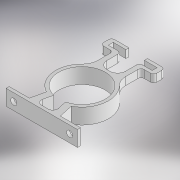
# Autodesk Inventor part: DefaultMotorMount
Saved by Autodesk Inventor 2018.2 (Build 222227000, 227)
## iProperties
Created: 2018-03-31
Part Number: DefaultMotorMount
Material: ABS Plastic
Document SubType Name: Modeling
Designer: Muchen He
Density: 1.06 g/cm^3
Appearance: Smooth - White
Author: Muchen He
Autodesk Inventor part; units mm, degrees
ref_plane "YZ Plane" through (0, 0, 0) normal (1, 0, 0) x (0, 1, 0)
ref_plane "XZ Plane" through (0, 0, 0) normal (0, 1, 0) x (-1, 0, 0)
ref_plane "XY Plane" through (0, 0, 0) normal (0, 0, 1) x (1, 0, 0)
sketch "Sketch1" plane through (0, 0, 0) normal (0, 0, 1) x (1, 0, 0)
  line L0 (0, 0) -> (23, 0)
  line L1 (23, 0) -> (23, 2)
  line L2 (23, 2) -> (10, 2)
  line L3 (10, 2) -> (8, 11)
  line L4 (0, 0) -> (0, 26) construction
  arc A0 (8, 11) -> (0, 43) centre (0, 26) ccw
  line L5 (18, 2) -> (18, 0) construction
  arc A1 (3.794, 11.4878) -> (0, 41) centre (0, 26) ccw
  line L6 (3.794, 11.4878) -> (5.0911, 5.6508)
  arc A2 (2.1626, 2) -> (5.0911, 5.6508) centre (2.1626, 5) ccw
  line L7 (2.1626, 2) -> (0, 2)
  line L8 (0, 0) -> (-23, 0)
  line L9 (-23, 0) -> (-23, 2)
  line L10 (-23, 2) -> (-10, 2)
  line L11 (-10, 2) -> (-8, 11)
  arc A3 (0, 43) -> (-8, 11) centre (0, 26) ccw
  arc A4 (0, 41) -> (-3.794, 11.4878) centre (0, 26) ccw
  line L12 (-3.794, 11.4878) -> (-5.0911, 5.6508)
  arc A5 (-5.0911, 5.6508) -> (-2.1626, 2) centre (-2.1626, 5) ccw
  line L13 (-2.1626, 2) -> (0, 2)
  dimension "d0" = 26
  dimension "d1" = 2
  dimension "d2" = 18
  dimension "d3" = 23
  dimension "d4" = 8
  dimension "d6" = 8
  dimension "d7" = 2
  dimension "d8" = 15
  dimension "d9" = 3
  dimension "d10" = 4
  constraints: 28 end point, 12 point on circle, 8 symmetric about line, 6 centre point, 4 perpendicular, 3 point on line, 2 tangent, 2 vertical alignment, 1 coincident, 1 concentric, 1 horizontal, 1 horizontal alignment, 1 vertical, 3 other
  measures "d0" distance of L0.start L4.end
  measures "d1" distance of L0.end L1.end
  measures "d2" distance between parallel lines of L4 L5
  measures "d3" distance between parallel lines of L4 L1
  measures "d4" distance from line of L5 L2.end
  measures "d6" distance from line of L4 L3.end
  measures "d7" radial gap between concentric circles of A1 A0
  measures "d8" radius of A1
  measures "d9" radius of A2
  measures "d10" distance between parallel lines of L3 L6
extrude "Extrusion1" add sketch "Sketch1" along normal blind 10
sketch "Sketch2" plane through (10, 2, 0) normal (0, 1, 0) x (1, 0, 0)
  line L0 (13, 0) -> (0, 0) projected
  line L1 (0, 0) -> (0, -10) projected
  line L2 (13, -10) -> (0, -10) projected
  line L3 (13, 0) -> (13, -10) projected
  line L4 (-20, 0) -> (-33, 0) projected
  line L5 (-33, 0) -> (-33, -10) projected
  line L6 (-20, -10) -> (-33, -10) projected
  line L7 (-20, 0) -> (-20, -10) projected
  circle A0 centre (-28, -5) radius 2
  circle A1 centre (8, -5) radius 2
  line L8 (-28, -5) -> (8, -5) construction
  point P0 (-10, 0)
  point P1 (-10, -5)
  point P2 (13, -5)
  point P3 (-33, -5)
  dimension "d13" = 36
  dimension "d14" = 4
  dimension "d15" = 4
  constraints: 3 midpoint, 2 centre point, 2 end point, 2 horizontal alignment, 1 horizontal, 1 vertical alignment
  measures "d13" distance of L8.start L8.end
  measures "d14" diameter of A1
  measures "d15" diameter of A0
extrude "Extrusion2" cut sketch "Sketch2" against normal up to next contours A0 | A1
sketch "Sketch3" plane through (0, 0, 10) normal (0, 0, 1) x (1, 0, 0)
  arc A0 (8, 11) -> (-8, 11) centre (0, 26) ccw projected
  line L0 (-6, 41.906) -> (-6, 57)
  line L1 (-6, 57) -> (-14.15, 57)
  line L2 (-14.15, 57) -> (-14.15, 60.2)
  line L3 (-14.15, 60.2) -> (-6, 60.2)
  line L4 (-6, 60.2) -> (-6, 62.2)
  line L5 (-6, 62.2) -> (-17.15, 62.2)
  line L6 (-17.15, 62.2) -> (-17.15, 55)
  line L7 (-17.15, 55) -> (-9, 55)
  line L8 (-9, 55) -> (-9, 40.4222)
  line L9 (0, 43) -> (0, 63.4755) construction
  point P0 (0, 0)
  dimension "d18" = 3.2
  dimension "d19" = 14.15
  dimension "d20" = 3
  dimension "d21" = 2
  dimension "d22" = 2
  dimension "d23" = 3
  dimension "d24" = 6
  dimension "d25" = 31
  constraints: 20 end point, 5 perpendicular, 4 vertical, 3 point on circle, 1 parallel, 1 point on line, 1 vertical alignment
  measures "d18" distance of L1.end L2.end
  measures "d19" distance between parallel lines of L2 L9
  measures "d20" distance between parallel lines of L2 L6
  measures "d21" distance between parallel lines of L5 L3
  measures "d22" distance between parallel lines of L1 L7
  measures "d23" distance between parallel lines of L0 L8
  measures "d24" distance between parallel lines of L9 L0
  measures "d25" distance from line of A0.centre L1
extrude "Extrusion3" add sketch "Sketch3" against normal blind 5
fillet "Fillet1" radius 2 4 edges at (-9, 55, 7.5) (-17.15, 55, 7.5) (-17.15, 62.2, 7.5) (-6, 57, 7.5)
fillet "Fillet1" radius 5 1 edges at (-6, 41.906, 7.5)
fillet "Fillet1" radius 10 1 edges at (-9, 40.4222, 7.5)
mirror "Mirror1" about plane through (0, 0, 0) normal (1, 0, 0) of "Extrusion3", "Fillet1"
body "Solid1"
